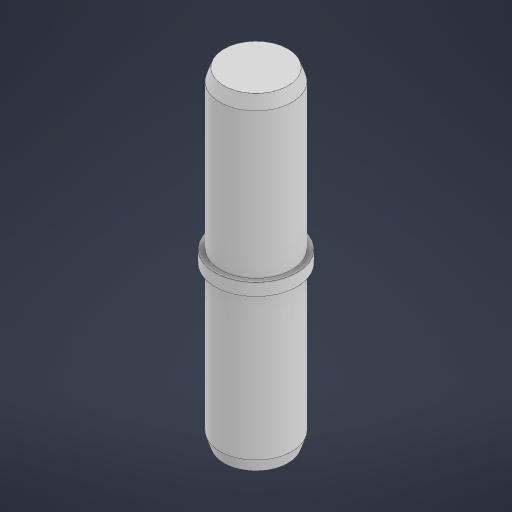
# Autodesk Inventor part: stange_verbinder
Saved by Autodesk Inventor 2023 (Build 270158000, 158)
## iProperties
Created: 2022-08-10
Part Number: stange_verbinder
Material: Generic
Document SubType Name: Modeling
Designer: bananenbrot
Density: 1 g/cm^3
Appearance: Default
Author: bananenbrot
Autodesk Inventor part; units mm, degrees
ref_plane "YZ Plane" through (0, 0, 0) normal (1, 0, 0) x (0, 1, 0)
ref_plane "XZ Plane" through (0, 0, 0) normal (0, 1, 0) x (-1, 0, 0)
ref_plane "XY Plane" through (0, 0, 0) normal (0, 0, 1) x (1, 0, 0)
sketch "Sketch2" plane through (0, 0, 0) normal (1, 0, 0) x (0, 1, 0)
  line L0 (0, 0) -> (59.3152, 0)
  line L1 (-40, 0) -> (40, 0)
  line L2 (40, 0) -> (40, -8.825)
  line L3 (40, -8.825) -> (-40, -8.825)
  line L4 (-40, -8.825) -> (-40, 0)
  line L5 (-1.5, -8.825) -> (1.5, -8.825)
  line L6 (1.5, -8.825) -> (1.5, -10.025)
  line L7 (1.5, -10.025) -> (-1.5, -10.025)
  line L8 (-1.5, -10.025) -> (-1.5, -8.825)
  point P0 (0, -10.025)
  point P1 (0, -8.825)
  dimension "d2" = 8.825
  dimension "d3" = 40
  dimension "d4" = 40
  dimension "d5" = 3
  dimension "d6" = 10.025
  constraints: 18 end point, 4 parallel, 3 horizontal, 3 midpoint, 2 perpendicular, 2 point on line, 1 vertical alignment
  measures "d2" distance of L3.end L1.start
  measures "d3" horizontal distance of L0.start L3.end
  measures "d4" horizontal distance of L0.start L2.end
  measures "d5" distance of L6.end L7.end
  measures "d6" distance from line of point (0, 0) L7
revolve "Revolution1" add sketch "Sketch2" angle 360 about axis through (0, 0, 0) along (0, 1, 0)
chamfer "Chamfer1" distance 1 distance2 3 1 edges at (0, 40, 8.825) measured on face at (2.071, 40, -2.6902)
chamfer "Chamfer2" distance 3 distance2 1 1 edges at (0, -40, 8.825) measured on face at (1.4156, -27.1667, -8.7107)
body "Solid1"
